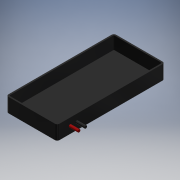
# Autodesk Inventor part: 739136_Holder
Saved by Autodesk Inventor 2017.1 (Build 211199000, 199)
## iProperties
Category: Electrical Accessories
Company: Autodesk Inc.
Created: 2014-11-27
Part Number: 739136_Holder
Material: Polystyrene, High Impact
Document SubType Name: Modeling
Designer: Tetrix
Density: 1.022 g/cm^3
Appearance: Smooth - Black
Catalog Web Link: http://www.tetrixrobotics.com/AA_Battery_Holder
Vendor: Tetrix
Author: Autodesk Inc.
Autodesk Inventor part; units mm, degrees
ref_plane "YZ Plane" through (0, 0, 0) normal (1, 0, 0) x (0, 1, 0)
ref_plane "XZ Plane" through (0, 0, 0) normal (0, 1, 0) x (-1, 0, 0)
ref_plane "XY Plane" through (0, 0, 0) normal (0, 0, 1) x (1, 0, 0)
sketch "Sketch1" plane through (0, 0, 0) normal (0, 1, 0) x (-1, 0, 0)
  line L0 (-57.15, -118.11) -> (-57.15, -2.54)
  arc A0 (-57.15, -118.11) -> (-54.61, -120.65) centre (-54.61, -118.11) ccw
  line L1 (-2.54, -120.65) -> (-54.61, -120.65)
  arc A1 (-2.54, -120.65) -> (0, -118.11) centre (-2.54, -118.11) ccw
  line L2 (0, -2.54) -> (0, -118.11)
  arc A2 (0, -2.54) -> (-2.54, 0) centre (-2.54, -2.54) ccw
  line L3 (-54.61, 0) -> (-2.54, 0)
  arc A3 (-54.61, 0) -> (-57.15, -2.54) centre (-54.61, -2.54) ccw
  point P0 (0, 0)
  point P1 (0, 0)
  constraints: 8 end point, 8 point on circle, 4 centre point
extrude "Extrusion1" add sketch "Sketch1" along normal blind 15.875
shell "Shell1" thickness 1.7 removed faces 1 at (38.1, 15.875, -41.0633)
sketch "Sketch2" plane through (57.15, 0, -2.54) normal (1, 0, 0) x (0, 0, -1)
  line L0 (0, 0) -> (115.57, 0) projected
  line L1 (115.57, 0) -> (115.57, 15.875) projected
  line L2 (0, 15.875) -> (115.57, 15.875) projected
  line L3 (0, 0) -> (0, 15.875) projected
  line L4 (118.11, 0) -> (118.11, 15.875) projected
  line L5 (-2.54, 0) -> (-2.54, 15.875) projected
  point P0 (11.96, 7.9375)
  point P1 (19.46, 7.9375)
  point P2 (0, 7.9375)
  dimension "d12" = 14.5
  dimension "d13" = 7.5
  constraints: 2 horizontal alignment, 1 midpoint
  measures "d12" distance from line of point (11.96, 7.938) L5
  measures "d13" distance of point (19.46, 7.938) point (11.96, 7.938)
hole "Hole2" at (57.15, 7.9375, -14.5) at (57.15, 7.9375, -22) direction (-1, 0, 0) diameter 3 end up to surface
sketch "Sketch4" plane through (57.15, 0, -2.54) normal (1, 0, 0) x (0, 0, -1)
  circle A0 centre (11.96, 7.9375) radius 1.5 projected
  circle A1 centre (19.46, 7.9375) radius 1.5 projected
  line L0 (0, 0) -> (115.57, 0) projected
  line L1 (115.57, 0) -> (115.57, 15.875) projected
  line L2 (0, 15.875) -> (115.57, 15.875) projected
  line L3 (0, 0) -> (0, 15.875) projected
  point P0 (-2.54, 0)
extrude "Extrusion2" add sketch "Sketch4" along normal blind 10 contours A0 | A1
body "Solid1"
